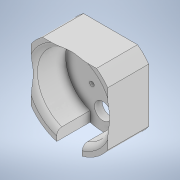
# Autodesk Inventor part: engine_cup
Saved by Autodesk Inventor 2020.1 (Build 241239000, 239)
## iProperties
Created: 2022-02-13
Part Number: engine_cup
Material: Generic
Document SubType Name: Modeling
Designer: OEM
Density: 1 g/cm^3
Appearance: Default
Author: OEM
Autodesk Inventor part; units mm, degrees
ref_plane "YZ Plane" through (0, 0, 0) normal (1, 0, 0) x (0, 1, 0)
ref_plane "XZ Plane" through (0, 0, 0) normal (0, 1, 0) x (-1, 0, 0)
ref_plane "XY Plane" through (0, 0, 0) normal (0, 0, 1) x (1, 0, 0)
sketch "Sketch1" plane through (0, 0, 0) normal (0, 0, 1) x (1, 0, 0)
  circle A0 centre (0, 0) radius 18.25 construction
  line L0 (12.904699, -12.904699) -> (-12.904699, 12.904699) construction
  line L1 (0, 29) -> (0, -41) construction
  line L2 (-75, 0) -> (78, 0) construction
  line L3 (-12.904699, -12.904699) -> (12.904699, 12.904699) construction
  line L4 (-12.904699, 12.904699) -> (12.904699, 12.904699) construction
  line L5 (12.904699, -12.904699) -> (12.904699, 12.904699) construction
  line L6 (-12.904699, -12.904699) -> (-12.904699, 12.904699) construction
  circle A1 centre (-4.242641, 4.242641) radius 0.9
  circle A2 centre (4.242641, 4.242641) radius 0.9
  circle A3 centre (-4.242641, -4.242641) radius 0.9
  circle A4 centre (4.242641, -4.242641) radius 0.9
  circle A5 centre (0, 0) radius 14.5
  line L7 (10.531498, 14.904699) -> (-10.531498, 14.904699)
  line L8 (-14.904699, 10.531498) -> (-14.904699, -10.531498)
  line L9 (14.904699, 10.531498) -> (14.904699, -10.531498)
  arc A6 (-10.531498, 14.904699) -> (-14.904699, 10.531498) centre (0, 0) ccw
  arc A7 (14.904699, 10.531498) -> (10.531498, 14.904699) centre (0, 0) ccw
  line L10 (-5, -13.610658) -> (-5, -17.551709)
  line L11 (5, -13.610658) -> (5, -17.551709)
  arc A8 (-14.904699, -10.531498) -> (-5, -17.551709) centre (0, 0) ccw
  arc A9 (5, -17.551709) -> (14.904699, -10.531498) centre (0, 0) ccw
  arc A10 (-5, -17.551709) -> (5, -17.551709) centre (0, 0) ccw
  circle A11 centre (0, -11.25) radius 3.25
  circle A12 centre (0, 0) radius 6 construction
  point P0 (5, -13.610658)
  point P1 (0, -14.5)
  point P2 (2.557391, -13.255556)
  point P3 (0, 0)
  dimension "d0" = 36.5
  dimension "d7" = 29
  dimension "d27" = 12
  dimension "d4" = 1.8
  dimension "d9" = 2
  dimension "d10" = 2
  dimension "d11" = 5
  dimension "d22" = 6.5
  dimension "d25" = 11.25
  dimension "d29" = 45
  constraints: 24 end point, 10 centre point, 10 point on circle, 9 symmetric about line, 6 coincident, 3 horizontal, 3 point on line, 2 midpoint, 2 perpendicular, 2 vertical, 20 other
  measures "d4" diameter of A1
  measures "d9" distance between parallel lines of L4 L7
  measures "d10" distance between parallel lines of L8 L6
  measures "d11" distance between parallel lines of L10 L1
  measures "d22" diameter of A11
  measures "d25" distance from line of L2 A11.centre
  measures "d29" angle of L2 L0
extrude "Extrusion1" add sketch "Sketch1" along normal blind 3 contours A11 | A5 | A5 L11 A10 L10
extrude "Extrusion2" add sketch "Sketch1" along normal blind 16 contours A5 L10 A8 L8 A6 L7 A7 L9 A9 L11
fillet "Fillet2" radius 1 4 edges at (3.3426, 4.2426, 0) (3.3426, -4.2426, 0) (-5.1426, -4.2426, 0) (-5.1426, 4.2426, 0)
extrude "Extrusion3" cut sketch "Sketch1" along normal blind 12 contours A11
fillet "Fillet3" radius 2 1 edges at (0, 14.5, 16)
body "Solid1"
